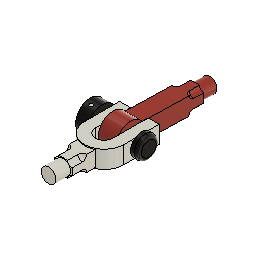
knuckle joint (Autodesk Fusion 360 design; units mm, degrees)
Autodesk Fusion 360 part; units mm, degrees
sketch "Sketch1" plane through (0, 0, 0) normal (0, 0, 1) x (1, 0, 0) in component "eye 1"
  circle A0 centre (0, 0) radius 10
  dimension "d1" = 20
  constraint coincident A0.centre origin
  measures "d1" diameter of A0
extrude "Extrude1" add sketch "Sketch1" along normal blind 20 makes body 1 in component "eye 1"
sketch "Sketch2" plane through (0, 0, 0) normal (1, 0, 0) x (0, 1, 0) in component "eye 1"
  line L0 (0, 0) -> (0, -100) construction
  circle A0 centre (0, -100) radius 10
  circle A1 centre (0, -100) radius 20
  dimension "d4" = 100
  dimension "d5" = 20
  dimension "d6" = 40
  constraint coincident L0.start origin
  constraint vertical L0
  constraint coincident L0.end A0.centre
  measures "d4" distance of L0.start L0.end
  measures "d5" diameter of A0
  measures "d6" diameter of A1
extrude "Extrude2" add sketch "Sketch2" along normal mid plane 24 separate body makes body 2 in component "eye 1"
sketch "Sketch3" plane through (0, 0, 0) normal (0, 0, -1) x (1, 0, 0) in component "eye 1"
  circle A0 centre (0, 0) radius 10
  line L0 (-12, 12) -> (12, 12)
  line L1 (12, 12) -> (12, -12)
  line L2 (12, -12) -> (-12, -12)
  line L3 (-12, -12) -> (-12, 12)
  line L4 (-12, 12) -> (12, -12) construction
  line L5 (12, 12) -> (-12, -12) construction
  dimension "d9" = 24
  constraint horizontal L0
  constraint perpendicular L0 L1
  constraint parallel L0 L2
  constraint parallel L1 L3
  constraint coincident L4 A0.centre
  constraint coincident L5 A0.centre
  constraint coincident A0.centre origin
  constraint equal L2 L3
  measures "d9" distance of L1.end L2.end
extrude "Extrude3" add sketch "Sketch3" along normal blind 85 contours A0 | L0 L1 L2 L3 bodies 1 2 in component "eye 1"
sketch "Sketch4" plane through (0, -12, 0) normal (0, -1, 0) x (1, 0, 0) in component "eye 1"
  line L0 (-12, -84) -> (12, -84)
  line L1 (12, -84) -> (12, 0)
  line L2 (12, 0) -> (-12, 0)
  line L3 (-12, 0) -> (-12, -84)
  line L4 (4.3907, 0) -> (12, 0)
  constraint coincident L2 L4.start
  constraint coincident L1.end L2.start
  constraint perpendicular L1 L4
sketch "Sketch5" plane through (0, -12, -42) normal (0, -1, 0) x (1, 0, 0) in component "eye 1"
  line L0 (12, 42) -> (6, 42)
  line L1 (6, 42) -> (6, 28)
  line L2 (12, -42) -> (12, 42)
  arc A0 (6, 28) -> (12, 22) centre (12, 28) ccw
  line L3 (12, 42) -> (-12, 42)
  point P0 (12, 42)
  point P1 (12, 42)
  dimension "d12" = 6
  dimension "d13" = 20
  dimension "d14" = 6
  constraint coincident P0 L0.start
  constraint perpendicular L0 L1
  constraint coincident L2 A0.end
  constraint tangent L1 A0
  measures "d12" distance of P1 L0.end
  measures "d13" distance of A0.end P1
  measures "d14" radius of A0
revolve "Revolve1" cut sketch "Sketch5" angle 360 about axis through (12, -12, -84) along (0, 0, 1) bodies 1 in component "eye 1"
mirror "Mirror1" about plane through (0, 0, 0) normal (0, 1, 0) of 2 faces at (6.0272, -11.4297, -9.3333) (7.0343, -8.7246, -14.7832) on bodies 1 in component "eye 1"
mirror "Mirror2" about plane through (0, 0, 0) normal (1, 0, 0) of 4 faces at (7.0343, 8.7246, -14.7832) (6.0272, 11.4297, -9.3333) (6.0272, -11.4297, -9.3333) (7.0343, -8.7246, -14.7832) on bodies 1 in component "eye 1"
sketch "Sketch1 (2)" plane through (0, 0, 0) normal (0, 0, 1) x (1, 0, 0) in component "fork end 1"
  circle A0 centre (0, 0) radius 10
  dimension "d20" = 20
  constraint coincident A0.centre origin
  measures "d20" diameter of A0
extrude "Extrude1'" add sketch "Sketch1 (2)" against normal blind 20 separate body makes body 3 in component "fork end 1"
sketch "Sketch4 (2)" plane through (0, 0, 0) normal (0, 1, 0) x (1, 0, 0) in component "fork end 1"
  line L0 (0, 0) -> (0, -80)
  line L1 (27, -104) -> (27, -56)
  arc A0 (27, -56) -> (-27, -56) centre (0, -56) ccw
  line L2 (-27, -56) -> (-27, -104)
  line L3 (-27, -104) -> (-12, -104)
  line L4 (-12, -104) -> (-12, -56)
  arc A1 (12, -56) -> (-12, -56) centre (0, -56) ccw
  line L5 (12, -104) -> (12, -56)
  line L6 (27, -104) -> (12, -104)
  dimension "d23" = 80
  dimension "d25" = 24
  dimension "d27" = 24
  dimension "d28" = 12
  dimension "d29" = 15
  constraint coincident L0.start origin
  constraint vertical L0
  constraint tangent L1 A0
  constraint tangent A0 L2
  constraint vertical L2
  constraint perpendicular L2 L3
  constraint perpendicular L3 L4
  constraint tangent L4 A1
  constraint tangent A1 L5
  constraint perpendicular L5 L6
  constraint collinear L3 L6
  constraint equal L2 L4
  constraint equal L1 L5
  constraint coincident A0.centre A1.centre
  constraint symmetric L0 L3.end L5.start
  measures "d23" distance of L0.start L0.end
  measures "d25" distance of L0.end L3
  measures "d27" distance of L0.end A0.centre
  measures "d28" radius of A1
  measures "d29" distance of L1.start L5.start
extrude "Extrude2'" add sketch "Sketch4 (2)" along normal mid plane 24 separate body makes body 4 in component "fork end 1"
sketch "Sketch5 (2)" plane through (0, 0, 0) normal (0, 0, 1) x (-1, 0, 0) in component "fork end 1"
  circle A0 centre (0, 0) radius 10
  line L0 (12, -10.6841) -> (-12, -10.6841)
  line L1 (-12, -10.6841) -> (-12, 10.6841)
  line L2 (-12, 10.6841) -> (12, 10.6841)
  line L3 (12, 10.6841) -> (12, -10.6841)
  line L4 (12, -10.6841) -> (-12, 10.6841) construction
  line L5 (-12, -10.6841) -> (12, 10.6841) construction
  dimension "d32" = 24
  constraint horizontal L0
  constraint perpendicular L0 L1
  constraint parallel L0 L2
  constraint parallel L1 L3
  constraint coincident L4 A0.centre
  constraint coincident L5 A0.centre
  constraint coincident A0.centre origin
  measures "d32" distance of L1.end L2.end
extrude "Extrude3'" add sketch "Sketch5 (2)" along normal blind 35 contours A0 | L0 L1 L2 L3 bodies 3 4 in component "fork end 1"
sketch "Sketch6" plane through (0, -10.6841, 0) normal (0, -1, 0) x (1, 0, 0) in component "fork end 1"
  arc A0 (-12, 31.8132) -> (12, 31.8132) centre (0, 56) ccw
  line L0 (-12, 31.8132) -> (-12, 0)
  line L1 (-12, 0) -> (12, 0)
  line L2 (12, 0) -> (12, 31.8132)
  line L3 (-12, 0) -> (-6, 0)
  line L4 (-6, 0) -> (-6, 14)
  line L5 (-12, 0) -> (-12, 20)
  arc A1 (-6, 14) -> (-12, 20) centre (-12, 14) ccw
  dimension "d35" = 6
  dimension "d36" = 20
  dimension "d37" = 6
  constraint coincident L0.end L1.start
  constraint perpendicular L0 L3
  constraint perpendicular L3 L4
  constraint coincident L0 L5.end
  constraint tangent L4 A1
  measures "d35" distance of L0.end L3.end
  measures "d36" distance of L0.end L5.end
  measures "d37" radius of A1
revolve "Revolve1'" cut sketch "Sketch6" angle 360 about axis through (-12, -10.6841, 31.8132) along (0, 0, -1) contours L0 L1 L3 L4 L5 A1 bodies 3 in component "fork end 1"
mirror "Mirror1'" about plane through (0, 0, 0) normal (0, 1, 0) of 2 faces at (-6.0272, -10.1137, 9.3333) (-7.0343, -7.4086, 14.7832) on bodies 3 in component "fork end 1"
mirror "Mirror2'" about plane through (0, 0, 0) normal (1, 0, 0) of 4 faces at (-6.0272, 10.1137, 9.3333) (-7.0343, 7.4086, 14.7832) (-6.0272, -10.1137, 9.3333) (-7.0343, -7.4086, 14.7832) on bodies 3 in component "fork end 1"
sketch "Sketch1 (3)" plane through (27, 0, 0) normal (1, 0, 0) x (0, 1, 0)
  line L0 (-12, 56) -> (12, 56)
  line L1 (12, 56) -> (12, 104)
  line L2 (12, 104) -> (-12, 104)
  line L3 (-12, 104) -> (-12, 56)
  circle A0 centre (0, 80) radius 10
  dimension "d43" = 20
  dimension "d44" = 12
  dimension "d45" = 24
  measures "d43" diameter of A0
  measures "d44" distance of L3 A0.centre
  measures "d45" distance of L2 A0.centre
extrude "Extrude4" cut sketch "Sketch1 (3)" against normal blind 54 contours A0 bodies 3 in component "fork end 1"
sketch "Sketch1 (4)" plane through (0, 0, 0) normal (0, 1, 0) x (1, 0, 0) in component "knuckle pin"
  circle A0 centre (0, 0) radius 10
  circle A1 centre (0, 0) radius 15
  dimension "d48" = 20
  dimension "d49" = 30
  constraint coincident A0.centre A1.centre
  measures "d48" diameter of A0
  measures "d49" diameter of A1
extrude "Extrude1''" add sketch "Sketch1 (4)" against normal blind 10 separate body contours A0 | A1 makes body 5 in component "knuckle pin"
extrude "Extrude2''" add sketch "Sketch1 (4)" along normal blind 70 contours A0 bodies 5 in component "knuckle pin"
fillet "Fillet1" radius 5 1 edges at (-13.9849, -10, -5.4242) on bodies 5 in component "knuckle pin"
sketch "Sketch2 (2)" plane through (0, 0, 0) normal (0, 0, 1) x (1, 0, 0) in component "knuckle pin"
  circle A0 centre (0, 62) radius 2
  line L0 (10, 70) -> (-10, 70)
  dimension "d56" = 4
  dimension "d57" = 8
  constraint vertical A0.centre origin
  measures "d56" diameter of A0
  measures "d57" distance of A0.centre L0
extrude "Extrude3''" cut sketch "Sketch2 (2)" along normal mid plane 20 bodies 5 in component "knuckle pin"
sketch "Sketch1 (5)" plane through (0, 0, 0) normal (0, 0, 1) x (1, 0, 0) in component "collar"
  circle A0 centre (0, 0) radius 10
  circle A1 centre (0, 0) radius 20
  dimension "d60" = 20
  dimension "d61" = 40
  constraint coincident A0.centre A1.centre
  measures "d60" diameter of A0
  measures "d61" diameter of A1
extrude "Extrude1'''" add sketch "Sketch1 (5)" against normal blind 16 separate body makes body 6 in component "collar"
sketch "Sketch2 (3)" plane through (0, 0, 0) normal (0, 1, 0) x (1, 0, 0) in component "collar"
  circle A0 centre (0, 8) radius 2
  line L0 (-20, 0) -> (20, 0)
  dimension "d64" = 4
  dimension "d65" = 8
  constraint vertical origin A0.centre
  measures "d64" diameter of A0
  measures "d65" distance of A0.centre L0
extrude "Extrude2'''" cut sketch "Sketch2 (3)" along normal mid plane 40 bodies 6 in component "collar"
sketch "Sketch1 (6)" plane through (0, 0, 0) normal (0, 0, 1) x (1, 0, 0) in component "pin"
  circle A0 centre (0, 0) radius 2
  dimension "d68" = 4
  constraint coincident A0.centre origin
  measures "d68" diameter of A0
ref_plane "WorkPlane1" through (0, 0, 40) normal (0, 0, 1) x (1, 0, 0) in component "pin"
sketch "Sketch2 (4)" plane through (0, 0, 40) normal (0, 0, 1) x (1, 0, 0) in component "pin"
  circle A0 centre (0, 0) radius 2.25
  dimension "d70" = 4.5
  constraint coincident A0.centre origin
  measures "d70" diameter of A0
loft "Loft1" add profiles "Sketch2 (4)", "Sketch1 (6)" section 1 section 2 separate body makes body 7 in component "pin"
move_body "Move1" bodies 3 to x (1, 0, 0) y (0, 1, 0) z (0, 0, 1) at (-43.6457, -36.6332, -6.5374) in component "fork end 1"
move_body "Move1'" bodies 6 to x (1, 0, 0) y (0, 1, 0) z (0, 0, 1) at (12, 66.81, -31.7163) in component "collar"
move_body "Move1''" bodies 1 to x (1, 0, 0) y (0, 1, 0) z (0, 0, 1) at (26.6216, -16.488, -43.1096) in component "eye 1"
move_body "Move2" bodies 3 to x (1, 0, 0) y (0, 0, -1) z (0, 1, 0) at (-43.9426, -133.8219, -44.9541) in component "fork end 1"
move_body "Move1'''" bodies 5 to x (-0.612781, 0.759016, 0.219985) y (-0.759016, -0.642788, 0.103531) z (0.219985, -0.103531, 0.969994) at (0, 0, 0) in component "knuckle pin"
component "knuckle pin" placed x (0.759016, -0.651072, 0) y (0.642788, 0.749358, 0.159016) z (-0.103531, -0.120695, 0.987276) at (-60.5882, -60.3593, -8.3208)
component "collar" placed x (0, -0.939693, -0.34202) y (0, 0.34202, -0.939693) z (1, 0, 0) at (-82.8719, -71.9333, 58.5643)
component "pin" placed x (0.778076, -0.591226, -0.212247) y (0.62817, 0.732317, 0.262898) z (0, -0.337881, 0.941189) at (-122.5882, -53.77, -26.6756)
component "eye 1" placed x (1, 0, 0) y (0, 1, 0) z (0, 0, 1) at (-114.2098, -43.8712, 134.7888)
component "fork end 1" placed x (1, 0, 0) y (0, 1, 0) z (0, 0, 1) at (0, 0, 0)
